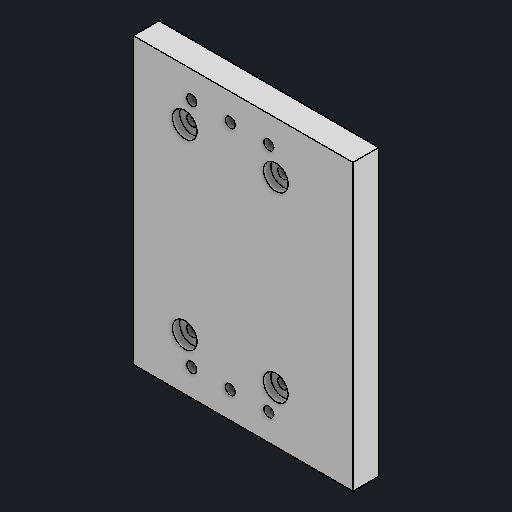
# Autodesk Inventor part: Adjustable Side Adapter Plate
Saved by Autodesk Inventor 2026.2 (Build 302298000, 298)
## iProperties
Created: 2026-04-18
Part Number: Adjustable Side Adapter Plate
Material: Generic
Document SubType Name: Modeling
Designer: JoshuaEah
Density: 1 g/cm^3
Appearance: Default
Author: JoshuaEah
Autodesk Inventor part; units mm, degrees
ref_plane "YZ Plane" through (0, 0, 0) normal (1, 0, 0) x (0, 1, 0)
ref_plane "XZ Plane" through (0, 0, 0) normal (0, 1, 0) x (-1, 0, 0)
ref_plane "XY Plane" through (0, 0, 0) normal (0, 0, 1) x (1, 0, 0)
sketch "Sketch1" plane through (0, 0, 0) normal (0, 0, 1) x (1, 0, 0)
  line L0 (0, 0) -> (83.1, 0)
  line L1 (83.1, 0) -> (83.1, 140.716)
  line L2 (83.1, 140.716) -> (0, 140.716)
  line L3 (0, 140.716) -> (0, 0)
  line L4 (83.1, 70.358) -> (0, 70.358)
  circle A0 centre (19.05, 115.358) radius 2.5
  circle A1 centre (19.05, 25.358) radius 2.5
  circle A2 centre (64.05, 115.358) radius 2.5
  circle A3 centre (64.05, 25.358) radius 2.5
  line L5 (41.55, 140.716) -> (41.55, 0)
  circle A4 centre (41.55, 127.508) radius 3.175
  circle A5 centre (41.55, 13.208) radius 3.175
  circle A6 centre (22.5, 127.508) radius 3.175
  circle A7 centre (22.5, 13.208) radius 3.175
  circle A8 centre (60.6, 127.508) radius 3.175
  circle A9 centre (60.6, 13.208) radius 3.175
  line L6 (83.1, 140.716) -> (102.15, 140.716)
  line L7 (102.15, 140.716) -> (102.15, 0)
  line L8 (102.15, 0) -> (83.1, 0)
  line L9 (83.1, 0) -> (83.1, 140.716)
  line L10 (0, 140.716) -> (-6.35, 140.716)
  line L11 (-6.35, 140.716) -> (-6.35, 0)
  line L12 (-6.35, 0) -> (0, 0)
  line L13 (0, 0) -> (0, 140.716)
  dimension "d0" = 140.716
  dimension "d1" = 5
  dimension "d2" = 90
  dimension "d3" = 19.05
  dimension "d6" = 45
  dimension "d11" = 19.05
  dimension "d12" = 6.35
  dimension "d13" = 114.3
  dimension "d32" = 19.05
  dimension "d37" = 19.05
  dimension "d38" = 6.35
  constraints: 28 end point, 10 centre point, 6 parallel, 5 horizontal, 4 midpoint, 3 perpendicular, 2 symmetric about line, 1 point on line, 14 other
  measures "d0" distance of L2.end L0.start
  measures "d1" diameter of A0
  measures "d2" diameter of A0.centre L4
  measures "d3" distance from line of L3 A0.centre
  measures "d6" distance of A0.centre A2.centre
  measures "d11" distance from line of L1 A2.centre
  measures "d12" diameter of A4
  measures "d13" diameter of A4.centre L4
  measures "d32" distance of A4.centre A6.centre
  measures "d37" distance of L1.end L6.end
  measures "d38" distance of L2.end L10.end
extrude "Extrusion1" add sketch "Sketch1" against normal blind 12.7 contours L3 L4 L5 A5 L0 | L12 L11 L10 L3 | L5 A5 L4 L1 L0 | L3 L2 L5 A4 L4 | L1 L6 L7 L8 | A5 L5 | L5 A5 | L5 A4 L2 L1 L4 | A4 L5 | L5 A4 | A0 | A1 | A2 | A3 | A6 | A7 | A8 | A9
hole "Hole1" at (19.05, 115.358, 0) at (64.05, 115.358, 0) at (64.05, 25.358, 0) at (19.05, 25.358, 0) direction (0, 0, -1) diameter 5.3086 end through all counterbore diameter 12.2428 counterbore depth 3.5814 clearance for "Hex Head Bolt" size "M5" standard "Ansi Metric M Profile"
hole "Hole2" at (22.5, 127.508, 0) at (60.6, 127.508, 0) at (22.5, 13.208, 0) at (60.6, 13.208, 0) at (41.55, 127.508, 0) at (41.55, 13.208, 0) direction (0, 0, -1) diameter 4.9784 end through all thread size "1/4-20 UNC" class "2B" standard "ANSI Unified Screw Threads"
equation "\"d11\" = d3"
body "Solid1"
